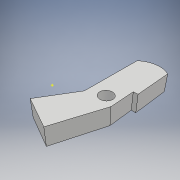
# Autodesk Inventor part: pin
Saved by Autodesk Inventor 2018 (Build 220112000, 112)
## iProperties
Created: 2020-12-04
Part Number: pin
Material: Všeobecné
Document SubType Name: Modeling
Designer: Jozko Mrkvicka
Density: 1 g/cm^3
Appearance: Výchozí
Author: Jozko Mrkvicka
Autodesk Inventor part; units mm, degrees
ref_plane "YZ Plane" through (0, 0, 0) normal (1, 0, 0) x (0, 1, 0)
ref_plane "XZ Plane" through (0, 0, 0) normal (0, 1, 0) x (-1, 0, 0)
ref_plane "XY Plane" through (0, 0, 0) normal (0, 0, 1) x (1, 0, 0)
sketch "Náčrt1" plane through (0, 0, 0) normal (0, 0, 1) x (1, 0, 0)
  arc A0 (17, 14) -> (10, 14) centre (13.5, 10) ccw
  circle A1 centre (13.5, 1) radius 1.5
  line L0 (16, 5.0055) -> (16, -0.6364)
  line L1 (16, 5.0055) -> (17, 5.0055)
  line L2 (17, 14) -> (17, 5.0055)
  line L3 (16, -0.6364) -> (12.2745, -10.872)
  line L4 (10, -0.6364) -> (10, 14)
  line L5 (5.3405, -8.3482) -> (10, -0.6364)
  line L6 (5.3405, -8.3482) -> (12.2745, -10.872)
  dimension "d65" = 3
  dimension "d70" = 9
  dimension "d71" = 1.6364
  constraints: 14 end point, 2 centre point, 2 horizontal alignment, 2 point on circle, 1 horizontal, 1 parallel, 1 vertical, 1 vertical alignment, 2 other
  measures "d65" diameter of A1
  measures "d70" distance of A1.centre A0.centre
  measures "d71" vertical distance of L4.start A1.centre
extrude "Vysunutí3" add sketch "Náčrt1" along normal blind 4
